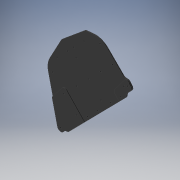
# Autodesk Inventor part: PlateRight
Saved by Autodesk Inventor 2019.3 (Build 233278000, 278)
## iProperties
Created: 2019-03-09
Part Number: PlateRight
Material: Generic
Document SubType Name: Modeling
Designer: eroldan
Density: 1 g/cm^3
Appearance: Default
Author: eroldan
Autodesk Inventor part; units mm, degrees
ref_plane "YZ Plane" through (0, 0, 0) normal (1, 0, 0) x (0, 1, 0)
ref_plane "XZ Plane" through (0, 0, 0) normal (0, 1, 0) x (-1, 0, 0)
ref_plane "XY Plane" through (0, 0, 0) normal (0, 0, 1) x (1, 0, 0)
sketch "Sketch1" plane through (0, 0, 0) normal (0, 0, 1) x (1, 0, 0)
  line L0 (163.9121, -54.1641) -> (147.5764, -34.4189)
  line L1 (147.5764, -34.4189) -> (132.6793, -34.0167)
  line L2 (132.6793, -34.0167) -> (55.1266, 43.4266)
  line L3 (55.1266, 43.4266) -> (0, 38.3883)
  line L4 (0, 38.3883) -> (-80.3007, -28.2671)
  line L5 (-130.7972, -122.1906) -> (-89.9473, -295.2085)
  line L6 (-80.3007, -28.2671) -> (-130.7972, -122.1906)
  circle A0 centre (-79.6232, -286.8257) radius 2.5 projected
  circle A1 centre (7.9154, -211.9549) radius 2.5 projected
  line L7 (142.9694, -75.2289) -> (163.9121, -54.1641)
  line L8 (142.9694, -75.2289) -> (140.1279, -88.6953)
  line L9 (140.1279, -88.6953) -> (-54.7034, -286.8257)
  line L10 (-54.7034, -286.8257) -> (-64.8995, -288.0349)
  line L11 (-64.8995, -288.0349) -> (-77.1232, -300.6747)
  line L12 (-77.1232, -300.6747) -> (-89.9473, -295.2085)
  circle A2 centre (42.9102, -176.2427) radius 2.5 projected
  circle A3 centre (88.0244, -130.2036) radius 2.5 projected
  circle A4 centre (123.0193, -94.4914) radius 2.5 projected
  circle A5 centre (135.5289, -57.202) radius 2.5 projected
  circle A6 centre (12.2005, -98.7604) radius 2.5 projected
  circle A7 centre (-28.3935, -140.1866) radius 2.5 projected
  circle A8 centre (-68.9875, -181.6128) radius 2.5 projected
  circle A9 centre (52.7945, -57.3343) radius 2.5 projected
  circle A10 centre (93.3885, -15.9081) radius 2.5 projected
  circle A11 centre (-111.1279, -140.3189) radius 2.5 projected
  circle A12 centre (-94.9802, -88.3546) radius 2.5 projected
  circle A13 centre (-59.9853, -52.6423) radius 2.5 projected
  circle A14 centre (-38.1892, -30.3994) radius 2.5 projected
  circle A15 centre (-3.1944, 5.3128) radius 2.5 projected
  circle A16 centre (51.2481, 25.3858) radius 2.5 projected
  circle A17 centre (-29.9399, -57.4666) radius 2.5 projected
  circle A18 centre (54.3409, -140.0543) radius 2.5 projected
  circle A19 centre (147.3739, -50.9497) radius 2.5 projected
  circle A20 centre (-26.8471, -222.9067) radius 2.5 projected
  point P0 (0, 0)
  constraints: 26 end point, 1 point on line
extrude "Extrusion1" add sketch "Sketch1" along normal blind 3
fillet "Fillet1" radius 60 2 edges at (55.1266, 43.4266, 1.5) (-130.7972, -122.1906, 1.5)
fillet "Fillet1" radius 10 11 edges at (-80.3007, -28.2671, 1.5) (0, 38.3883, 1.5) (147.5764, -34.4189, 1.5) (132.6793, -34.0167, 1.5) (163.9121, -54.1641, 1.5) (142.9694, -75.2289, 1.5) (140.1279, -88.6953, 1.5) (-54.7034, -286.8257, 1.5) (-64.8995, -288.0349, 1.5) (-77.1232, -300.6747, 1.5) (-89.9473, -295.2085, 1.5)
sketch "Sketch2" plane through (0, 0, 3) normal (0, 0, 1) x (1, 0, 0)
  line L0 (-125.5671, -144.3425) -> (-91.1088, -290.2891) projected
  arc A0 (-91.1088, -290.2891) -> (-85.2975, -297.1904) centre (-81.3764, -287.9913) ccw projected
  arc A1 (-83.4509, -297.9775) -> (-72.3414, -295.7301) centre (-79.5298, -288.7784) ccw projected
  line L1 (-85.2975, -297.1904) -> (-83.4509, -297.9775) projected
  line L2 (-72.3414, -295.7301) -> (-67.3746, -290.5943) projected
  arc A2 (-61.3639, -287.6156) -> (-67.3746, -290.5943) centre (-60.1862, -297.546) ccw projected
  line L3 (-61.3639, -287.6156) -> (-58.1924, -287.2395) projected
  arc A3 (-58.1924, -287.2395) -> (-52.2399, -284.3205) centre (-59.3701, -277.3091) ccw projected
  line L4 (-52.2399, -284.3205) -> (138.0773, -90.7806) projected
  line L5 (-52.2399, -284.3205) -> (138.0773, -90.7806) projected
  line L6 (0, -231.196) -> (-68.9875, -159.1175)
  circle A4 centre (-68.9875, -181.6128) radius 2.5 projected
  line L7 (-68.9875, -159.1175) -> (-109.8238, -211.0225)
  circle A5 centre (-26.8471, -222.9067) radius 2.5 projected
  circle A6 centre (-79.6232, -286.8257) radius 2.5 projected
  point P0 (0, 0)
  constraints: 4 end point, 2 point on line
extrude "Extrusion2" add sketch "Sketch2" along normal blind 3 separate body
fillet "Fillet2" radius 10 1 edges at (-68.9875, -159.1175, 4.5)
sketch "Sketch3" plane through (0, 0, 3) normal (0, 0, 1) x (1, 0, 0)
  line L0 (129.8625, -31.2039) -> (75.0063, 23.575) projected
  arc A0 (129.8625, -31.2039) -> (136.6587, -34.1242) centre (136.9286, -24.1278) ccw projected
  line L1 (143.0364, -34.2963) -> (136.6587, -34.1242) projected
  arc A1 (150.4715, -37.9182) -> (143.0364, -34.2963) centre (142.7665, -44.2927) ccw projected
  line L2 (158.1285, -47.1734) -> (150.4715, -37.9182) projected
  arc A2 (157.5152, -60.5983) -> (158.1285, -47.1734) centre (150.4236, -53.5479) ccw projected
  line L3 (145.0524, -73.1338) -> (157.5152, -60.5983) projected
  arc A3 (145.0524, -73.1338) -> (142.3595, -78.1196) centre (152.144, -80.1842) ccw projected
  line L4 (140.7317, -85.8338) -> (142.3595, -78.1196) projected
  arc A4 (138.0773, -90.7806) -> (140.7317, -85.8338) centre (130.9471, -83.7691) ccw projected
  line L5 (-52.2399, -284.3205) -> (138.0773, -90.7806) projected
  line L6 (119.0571, -110.1229) -> (98.7577, -88.4973)
  line L7 (98.7577, -88.4973) -> (139.8475, -34.2102)
  circle A5 centre (123.0193, -94.4914) radius 2.5 projected
  circle A6 centre (135.5289, -57.202) radius 2.5 projected
  circle A7 centre (147.3739, -50.9497) radius 2.5 projected
  point P0 (0, 0)
  constraints: 4 end point, 1 midpoint, 1 point on line
extrude "Extrusion3" add sketch "Sketch3" along normal blind 3 separate body
fillet "Fillet3" radius 10 1 edges at (98.7577, -88.4973, 4.5)
